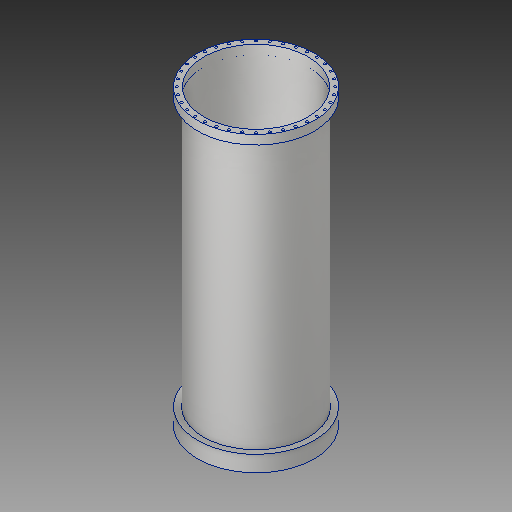
# Autodesk Inventor part: Radiation Sheild 2K
Saved by Autodesk Inventor 2018 (Build 220112000, 112)
## iProperties
Created: 2018-10-10
Part Number: Radiation Sheild 2K
Material: Generic
Document SubType Name: Modeling
Designer: Admin
Density: 1 g/cm^3
Appearance: Aluminum - Flat
Author: Admin
Autodesk Inventor part; units mm, degrees
note: some values were not read from the file. Chosen so that the rebuilt part matches the saved one: direction of "Hole1".
ref_plane "YZ Plane" through (0, 0, 0) normal (1, 0, 0) x (0, 1, 0)
ref_plane "XZ Plane" through (0, 0, 0) normal (0, 1, 0) x (-1, 0, 0)
ref_plane "XY Plane" through (0, 0, 0) normal (0, 0, 1) x (1, 0, 0)
sketch "Sketch1" plane through (0, 0, 0) normal (0, 1, 0) x (-1, 0, 0)
  circle A0 centre (0, 0) radius 161.925
  circle A1 centre (0, 0) radius 144.4625
  dimension "d0" = 323.85
  dimension "d1" = 288.925
  constraints: 2 centre point, 2 coincident
  measures "d0" diameter of A0
  measures "d1" diameter of A1
extrude "Extrusion1" add sketch "Sketch1" along normal blind 25.4
sketch "Sketch2" plane through (0, 0, 0) normal (0, -1, 0) x (1, 0, 0)
  circle A0 centre (0, 0) radius 144.4625
  circle A1 centre (0, 0) radius 146.05
  dimension "d4" = 288.925
  dimension "d5" = 292.1
  constraints: 2 centre point, 2 coincident
  measures "d4" diameter of A0
  measures "d5" diameter of A1
extrude "Extrusion2" add sketch "Sketch2" along normal blind 742.95
sketch "Sketch3" plane through (0, -742.95, 0) normal (0, -1, 0) x (1, 0, 0)
  circle A0 centre (0, 0) radius 144.4625
  circle A1 centre (0, 0) radius 161.925
  dimension "d8" = 288.925
  dimension "d9" = 323.85
  constraints: 2 centre point, 2 coincident
  measures "d8" diameter of A0
  measures "d9" diameter of A1
extrude "Extrusion3" add sketch "Sketch3" along normal blind 25.4
sketch "Sketch4" plane through (0, -768.35, 0) normal (0, -1, 0) x (1, 0, 0)
  circle A0 centre (0, 0) radius 161.925
  dimension "d12" = 323.85
  constraints: 1 centre point, 1 coincident
  measures "d12" diameter of A0
extrude "Extrusion4" add sketch "Sketch4" along normal blind 19.05
sketch "Sketch5" plane through (0, 25.4, 0) normal (0, 1, 0) x (1, 0, 0)
  line L0 (0, 0) -> (154.983, 13.5593)
  line L1 (0, 0) -> (155.575, 0) construction
  dimension "d15" = 155.575
  dimension "d16" = 5
  constraints: 4 end point, 1 equal length, 1 horizontal
  measures "d15" distance of L0.start L0.end
  measures "d16" angle of L1 L0
hole "Hole1" at (154.983, 25.4, -13.5593) direction (0, -1, 0) diameter 6.7564 end up to surface clearance for "Flat Head Machine Screw (82)" size "1/4" standard "Ansi Unified Screw Threads"
pattern_circular "Circular Pattern1" count 36 over 360 about axis through (0, 0, 0) along (0, -1, 0) of "Hole1"
body "Solid1"
